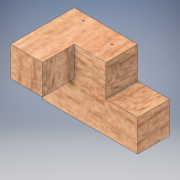
# Autodesk Inventor part: Ied Final
Saved by Autodesk Inventor 2018 (Build 220112000, 112)
## iProperties
Created: 2019-06-10
Part Number: Ied Final
Material: Generic
Document SubType Name: Modeling
Designer: 10043883
Density: 1 g/cm^3
Appearance: Birch - Natural Polished
Author: 10043883
Autodesk Inventor part; units mm, degrees
ref_plane "YZ Plane" through (0, 0, 0) normal (1, 0, 0) x (0, 1, 0)
ref_plane "XZ Plane" through (0, 0, 0) normal (0, 1, 0) x (-1, 0, 0)
ref_plane "XY Plane" through (0, 0, 0) normal (0, 0, 1) x (1, 0, 0)
sketch "Sketch1" plane through (0, 0, 0) normal (0, 0, 1) x (1, 0, 0)
  line L0 (18.5864, 6.043) -> (94.7864, 6.043)
  line L1 (94.7864, 6.043) -> (94.7864, -44.757)
  line L2 (94.7864, -44.757) -> (18.5864, -44.757)
  line L3 (18.5864, -44.757) -> (18.5864, 6.043)
  point P0 (0, 0)
  dimension "d0" = 76.2
  dimension "d1" = 50.8
  constraints: 8 end point, 2 parallel, 1 horizontal, 1 perpendicular
  measures "d0" distance of L1.end L2.end
  measures "d1" distance of L0.end L1.end
extrude "Extrusion1" add sketch "Sketch1" along normal blind 50.8
sketch "Sketch2" plane through (94.7864, -44.757, 0) normal (1, 0, 0) x (0, 0, -1)
  line L0 (0, 50.8) -> (-50.8, 50.8) projected
  line L1 (0, 0) -> (-50.8, 0) projected
  line L2 (-50.8, 50.8) -> (-25.4, 50.8)
  line L3 (-25.4, 50.8) -> (-25.4, 0)
  line L4 (-25.4, 0) -> (-50.8, 0)
  line L5 (-50.8, 0) -> (-50.8, 50.8)
  point P0 (0, 44.757)
  dimension "d4" = 25.4
  constraints: 8 end point, 2 parallel, 1 horizontal, 1 midpoint, 1 perpendicular
  measures "d4" distance of L3.end L4.end
extrude "Extrusion2" cut sketch "Sketch2" against normal blind 50.8
sketch "Sketch3" plane through (18.5864, -44.757, 0) normal (-1, 0, 0) x (0, 0, 1)
  point P0 (0, 44.757)
sketch "Sketch4" plane through (18.5864, -44.757, 0) normal (-1, 0, 0) x (0, 0, 1)
  line L0 (0, 0) -> (50.8, 0) projected
  line L1 (50.8, 0) -> (25.4, 0)
  line L2 (25.4, 0) -> (25.4, 26.8957)
  line L3 (25.4, 26.8957) -> (50.8, 26.8957)
  line L4 (50.8, 26.8957) -> (50.8, 0)
  point P0 (0, 44.757)
  dimension "d7" = 25.4
  constraints: 8 end point, 2 parallel, 1 horizontal, 1 perpendicular
  measures "d7" distance of L2.end L3.end
extrude "Extrusion3" cut sketch "Sketch4" against normal blind 50.8
sketch "Sketch5" plane through (94.7864, -44.757, 25.4) normal (0, 0, 1) x (1, 0, 0)
  line L0 (-50.8, 50.8) -> (0, 50.8) projected
  line L1 (0, 50.8) -> (-25.4, 50.8)
  line L2 (-25.4, 50.8) -> (-25.4, 25.4)
  line L3 (-25.4, 25.4) -> (0, 25.4)
  line L4 (0, 25.4) -> (0, 50.8)
  point P0 (-94.7864, 44.757)
  dimension "d10" = 25.4
  dimension "d11" = 25.4
  constraints: 8 end point, 2 parallel, 1 horizontal, 1 perpendicular
  measures "d10" distance of L3.end L2.end
  measures "d11" distance of L2.end L1.end
extrude "Extrusion4" cut sketch "Sketch5" against normal blind 50.8
body "Solid1"
